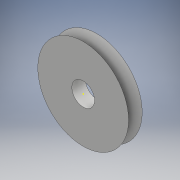
# Autodesk Inventor part: Wrist polley
Saved by Autodesk Inventor 2018 (Build 220112000, 112)
## iProperties
Created: 2018-02-08
Part Number: Wrist polley
Material: Générique
Document SubType Name: Modeling
Designer: Thomas
Density: 1 g/cm^3
Appearance: Par défaut
Author: Thomas
Autodesk Inventor part; units mm, degrees
ref_plane "YZ Plane" through (0, 0, 0) normal (1, 0, 0) x (0, 1, 0)
ref_plane "XZ Plane" through (0, 0, 0) normal (0, 1, 0) x (-1, 0, 0)
ref_plane "XY Plane" through (0, 0, 0) normal (0, 0, 1) x (1, 0, 0)
sketch "Esquisse1" plane through (0, 0, 0) normal (0, 0, 1) x (1, 0, 0)
  point P0 (0, 0)
sketch "Esquisse2" plane through (0, 0, 0) normal (0, 0, 1) x (1, 0, 0)
  line L0 (0, 2.5) -> (14.5, 2.5)
  line L1 (14.5, 2.5) -> (20, 0)
  line L2 (20, 0) -> (0, 0)
  line L3 (0, 0) -> (0, 2.5)
  dimension "d0" = 20
  dimension "d1" = 14.5
  dimension "d2" = 2.5
  constraints: 8 end point, 1 horizontal, 1 parallel, 1 perpendicular
  measures "d0" distance of L1.end L2.end
  measures "d1" distance of L0.start L0.end
  measures "d2" distance of L2.end L0.start
revolve "Révolution1" add sketch "Esquisse2" angle 360 about axis through (0, 0, 0) along (0, 1, 0)
sketch "Esquisse3" plane through (0, 0, 0) normal (0, 0, 1) x (1, 0, 0)
  line L0 (-14.5, 2.5) -> (14.5, 2.5) projected
  line L1 (0, 2.5) -> (14.5, 2.5)
  line L2 (14.5, 2.5) -> (14.5, 3.5)
  line L3 (14.5, 3.5) -> (0, 3.5)
  line L4 (0, 3.5) -> (0, 2.5)
  point P0 (0, 0)
  dimension "d4" = 1
  dimension "d5" = 14.5
  constraints: 8 end point, 2 parallel, 1 horizontal, 1 midpoint, 1 perpendicular
  measures "d4" distance of L1.end L2.end
  measures "d5" distance of L2.end L3.end
revolve "Révolution2" add sketch "Esquisse3" angle 360 about axis through (0, 3.5, 0) along (0, -1, 0)
sketch "Esquisse4" plane through (0, 0, 0) normal (0, 0, 1) x (1, 0, 0)
  line L0 (-14.5, 3.5) -> (14.5, 3.5) projected
  line L1 (0, 3.5) -> (0, 6)
  line L2 (0, 6) -> (20, 6)
  line L3 (20, 6) -> (14.5, 3.5)
  line L4 (14.5, 3.5) -> (0, 3.5)
  point P0 (0, 0)
  dimension "d7" = 20
  dimension "d8" = 2.5
  constraints: 8 end point, 1 collinear, 1 midpoint, 1 perpendicular, 1 vertical
  measures "d7" distance of L1.end L2.end
  measures "d8" distance of L1.start L1.end
revolve "Révolution3" add sketch "Esquisse4" angle 360 about axis through (0, 3.5, 0) along (0, 1, 0)
sketch "Esquisse5" plane through (0, 6, 0) normal (0, 1, 0) x (1, 0, 0)
  circle A0 centre (0, 0) radius 5
  dimension "d10" = 10
  constraints: 1 centre point, 1 coincident
  measures "d10" diameter of A0
extrude "Extrusion1" cut sketch "Esquisse5" against normal blind 6
